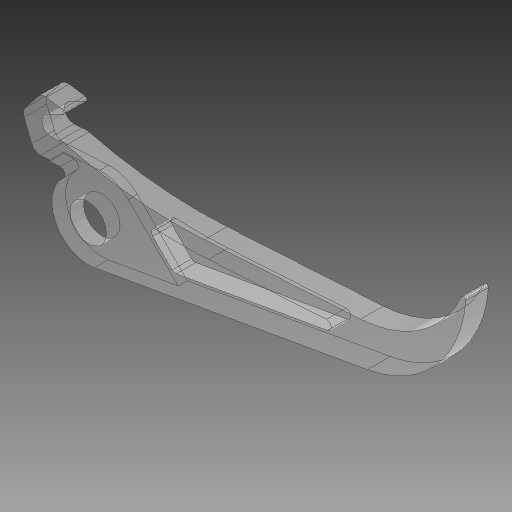
# Autodesk Inventor part: 後ウイング1.2
Saved by Autodesk Inventor 2020 (Build 240168000, 168)
## iProperties
Created: 2019-09-05
Part Number: 後ウイング1.2
Material: ポリカーボネート、クリア
Document SubType Name: Modeling
Designer: 雪村
Density: 1.2 g/cm^3
Appearance: ポリカーボネート - クリア
Mass: 5.3588 g
Surface Area: 38.9825 cm^2
Volume: 4.46567 cm^3
Description: ポリカ 5t
Author: 雪村
Autodesk Inventor part; units mm, degrees
ref_plane "YZ Plane" through (0, 0, 0) normal (1, 0, 0) x (0, 1, 0)
ref_plane "XZ Plane" through (0, 0, 0) normal (0, 1, 0) x (-1, 0, 0)
ref_plane "XY Plane" through (0, 0, 0) normal (0, 0, 1) x (1, 0, 0)
sketch "スケッチ1" plane through (0, 0, 0) normal (0, 0, 1) x (1, 0, 0)
  circle A0 centre (243.856358, 111.9666) radius 4.025
  circle A1 centre (243.856358, 111.9666) radius 8
  line L0 (245.245543, 104.088138) -> (305.438145, 114.701717)
  line L1 (243.379474, 119.952373) -> (303.875311, 123.564987)
  line L2 (243.856358, 111.9666) -> (322.640978, 125.858454) construction
  arc A2 (305.438145, 114.701717) -> (327.084101, 138.703402) centre (300.875427, 140.578172) ccw
  arc A3 (303.875311, 123.564987) -> (326.129046, 138.943438) centre (302.320232, 149.605909) ccw
  circle A4 centre (326.585375, 138.739077) radius 0.5
  line L3 (305.438145, 114.701717) -> (330.058338, 119.042922) construction
  line L4 (330.058338, 119.042922) -> (326.585375, 138.739077) construction
  line L5 (305.438145, 114.701717) -> (303.875311, 123.564987) construction
  point P0 (0, 0)
  point P1 (0, 0)
  dimension "d1" = 1
  dimension "d2" = 20
  dimension "d3" = 9
  dimension "d4" = 25
  dimension "d7" = 16
  dimension "d8" = 8.05
  constraints: 12 end point, 9 point on circle, 6 tangent, 5 centre point, 2 parallel, 2 perpendicular, 3 other
  measures "d1" diameter of A4
  measures "d2" distance of L3.end L4.end
  measures "d3" distance from line of L1.end L0
  measures "d4" distance of L0.end L3.end
  measures "d7" diameter of A1
  measures "d8" diameter of A0
extrude "押し出し1" add sketch "スケッチ1" along normal blind 5
sketch "スケッチ3" plane through (0, 0, 0) normal (0, 0, -1) x (-1, 0, 0)
  circle A0 centre (-243.856358, 111.9666) radius 4.025
  arc A1 (-326.129046, 138.943438) -> (-303.875311, 123.564987) centre (-302.320232, 149.605909) ccw
  arc A2 (-326.129046, 138.943438) -> (-327.084101, 138.703402) centre (-326.585375, 138.739077) ccw
  arc A3 (-327.084101, 138.703402) -> (-305.438145, 114.701717) centre (-300.875427, 140.578172) ccw
  line L0 (-245.245543, 104.088138) -> (-305.438145, 114.701717)
  arc A4 (-245.245543, 104.088138) -> (-243.379474, 119.952373) centre (-243.856358, 111.9666) ccw
  line L1 (-303.875311, 123.564987) -> (-243.379474, 119.952373)
  circle A5 centre (-243.856358, 111.9666) radius 4.025
  circle A6 centre (-243.856358, 111.9666) radius 8.25
  point P0 (0, 0)
  point P1 (-243.432312, 120.205695)
  point P2 (-245.288956, 103.841936)
  point P3 (-247.230487, 104.438137)
  point P4 (-245.391454, 120.072522)
  dimension "d9" = 16.5
  constraints: 1 centre point, 1 coincident
  measures "d9" diameter of A6
extrude "押し出し2" cut sketch "スケッチ3" against normal blind 2 contours A6 L0 A4 L1 | L1 A4 L0 A6
sketch "スケッチ4" plane through (0, 0, 5) normal (0, 0, 1) x (1, 0, 0)
  line L0 (303.875311, 123.564987) -> (245.391454, 120.072522)
  line L1 (245.391454, 120.072522) -> (235.409237, 119.476417)
  line L2 (235.409237, 119.476417) -> (235.051458, 125.467679)
  arc A0 (235.051458, 125.467679) -> (269.471333, 121.510494) centre (263.510279, 221.332665) ccw
  circle A1 centre (243.856358, 111.9666) radius 4.025
  circle A2 centre (237.755765, 122.120997) radius 2.5
  point P0 (0, 0)
  point P1 (0, 0)
  dimension "d44" = 5
  dimension "d45" = 100
  dimension "d46" = 10
  constraints: 4 end point, 4 tangent, 2 centre point, 2 point on circle, 1 collinear, 1 perpendicular, 1 point on line
  measures "d44" diameter of A2
  measures "d45" radius of A0
  measures "d46" distance of L0.end L1.end
extrude "押し出し3" add sketch "スケッチ4" against normal blind 5 contours L0 L1 A2 A0 | A2 L2 A0 | A2 | L1 L2 A2
sketch "スケッチ5" plane through (0, 0, 0) normal (0, 0, -1) x (-1, 0, 0)
  circle A0 centre (-243.856358, 111.9666) radius 4.025
  circle A1 centre (-243.856358, 111.9666) radius 8.25
  line L0 (-249.689989, 117.800231) -> (-288.164279, 79.32594)
  line L1 (-247.230487, 104.438137) -> (-305.438145, 114.701717)
  point P0 (0, 0)
  point P1 (-260.730499, 106.75972)
  point P2 (-245.288956, 103.841936)
  point P3 (-260.840494, 106.649726)
  point P4 (-260.680485, 106.809734)
  dimension "d35" = 16.5
  dimension "d36" = 55
  constraints: 2 end point, 1 centre point, 1 coincident, 1 point on circle, 1 tangent, 1 other
  measures "d35" diameter of A1
extrude "押し出し4" cut sketch "スケッチ5" against normal blind 2 contours A1 L1 L0
fillet "フィレット3" radius 3 1 edges at (235.0515, 125.4677, 2.5)
sketch "スケッチ6" plane through (0, 0, 5) normal (0, 0, 1) x (1, 0, 0)
  line L0 (245.391454, 120.072522) -> (243.379474, 119.952373)
  arc A0 (239.030137, 124.375341) -> (235.301068, 121.28779) centre (238.295733, 121.466622) ccw
  line L1 (235.301068, 121.28779) -> (235.409237, 119.476417)
  line L2 (235.409237, 119.476417) -> (243.379474, 119.952373)
  arc A1 (243.379474, 119.952373) -> (245.245543, 104.088138) centre (243.856358, 111.9666) ccw
  line L3 (245.245543, 104.088138) -> (305.438145, 114.701717)
  arc A2 (305.438145, 114.701717) -> (327.084101, 138.703402) centre (300.875427, 140.578172) ccw
  arc A3 (327.084101, 138.703402) -> (326.129046, 138.943438) centre (326.585375, 138.739077) ccw
  arc A4 (303.875311, 123.564987) -> (326.129046, 138.943438) centre (302.320232, 149.605909) ccw
  line L4 (303.875311, 123.564987) -> (269.471333, 121.510494)
  arc A5 (239.030137, 124.375341) -> (269.471333, 121.510494) centre (263.510279, 221.332665) ccw
  circle A6 centre (243.856358, 111.9666) radius 4.025
  circle A7 centre (237.79229, 118.616943) radius 1
  arc A8 (243.379474, 119.952373) -> (245.245543, 104.088138) centre (243.856358, 111.9666) ccw
  line L5 (235.409237, 119.476417) -> (243.379474, 119.952373)
  line L6 (235.301068, 121.28779) -> (235.409237, 119.476417)
  point P0 (0, 0)
  point P1 (236.794068, 118.557333)
  point P2 (238.466075, 117.878016)
  point P3 (237.732679, 119.615165)
  point P4 (237.732679, 119.615165)
  dimension "d55" = 2
  constraints: 5 other
extrude "押し出し5" add sketch "スケッチ6" against normal up to surface (3 mm away) contours A5 L4 A4 A3 A2 L3 A1 L2 L1 A0 | L2 A1 A7
sketch "スケッチ7" plane through (0, 0, 0) normal (0, 0, -1) x (-1, 0, 0)
  line L0 (-245.391454, 120.072522) -> (-235.409237, 119.476417)
  arc A0 (-245.391454, 120.072522) -> (-249.689989, 117.800231) centre (-243.856358, 111.9666) ccw
  line L1 (-260.680485, 106.809734) -> (-249.689989, 117.800231)
  circle A1 centre (-243.856358, 111.9666) radius 8.25
  line L2 (-243.364571, 120.201929) -> (-235.394334, 119.725972)
  line L3 (-235.409237, 119.476417) -> (-235.490786, 118.110823)
  arc A2 (-235.784063, 117.342881) -> (-236.275398, 114.521799) centre (-233.432538, 115.479999) ccw
  arc A3 (-238.466075, 117.878016) -> (-237.732679, 119.615165) centre (-237.79229, 118.616943) ccw
  line L4 (-235.409237, 119.476417) -> (-235.301068, 121.28779)
  point P0 (0, 0)
  point P1 (-249.689989, 117.800231)
  point P2 (-241.367494, 119.832224)
  dimension "d52" = 16.5
  constraints: 2 end point, 1 coincident, 1 parallel, 1 point on line, 4 other
extrude "押し出し6" cut sketch "スケッチ7" against normal blind 2 contours L0 A1 L2 L4 | A1 A0 L0 | L0 A1
sketch "スケッチ8" plane through (0, 0, 0) normal (0, 0, -1) x (-1, 0, 0)
  arc A0 (-243.364571, 120.201929) -> (-249.689989, 117.800231) centre (-243.856358, 111.9666) ccw
  line L0 (-243.364571, 120.201929) -> (-235.394334, 119.725972)
  line L1 (-235.394334, 119.725972) -> (-235.301068, 121.28779)
  arc A1 (-235.301068, 121.28779) -> (-239.030137, 124.375341) centre (-238.295733, 121.466622) ccw
  arc A2 (-269.471333, 121.510494) -> (-239.030137, 124.375341) centre (-263.510279, 221.332665) ccw
  line L2 (-303.875311, 123.564987) -> (-269.471333, 121.510494)
  arc A3 (-326.129046, 138.943438) -> (-303.875311, 123.564987) centre (-302.320232, 149.605909) ccw
  arc A4 (-326.129046, 138.943438) -> (-327.084101, 138.703402) centre (-326.585375, 138.739077) ccw
  arc A5 (-327.084101, 138.703402) -> (-305.438145, 114.701717) centre (-300.875427, 140.578172) ccw
  line L3 (-260.680485, 106.809734) -> (-305.438145, 114.701717)
  line L4 (-260.680485, 106.809734) -> (-249.689989, 117.800231)
  arc A6 (-235.68768, 124.269668) -> (-234.722388, 128.05367) centre (-235.624481, 126.268669) ccw
  line L5 (-232.816946, 130.554466) -> (-230.034777, 127.017584)
  arc A7 (-232.816946, 130.554466) -> (-234.673777, 131.297553) centre (-234.388893, 129.317947) ccw
  line L6 (-234.722388, 128.05367) -> (-238.29239, 129.857855)
  line L7 (-238.138088, 130.799007) -> (-234.673777, 131.297553)
  line L8 (-233.397891, 119.606751) -> (-235.394334, 119.725972)
  arc A8 (-233.397891, 119.606751) -> (-231.421838, 120.860108) centre (-233.27867, 121.603195) ccw
  line L9 (-229.749893, 125.037978) -> (-231.421838, 120.860108)
  arc A9 (-229.749893, 125.037978) -> (-230.034777, 127.017584) centre (-231.606724, 125.781065) ccw
  line L10 (-239.030137, 124.375341) -> (-235.68768, 124.269668)
  arc A10 (-238.138088, 130.799007) -> (-238.29239, 129.857855) centre (-238.066867, 130.304105) ccw
  line L11 (-235.394334, 119.725972) -> (-239.030137, 124.375341)
  line L12 (-235.394334, 119.725972) -> (-239.030137, 124.375341)
  arc A11 (-235.301068, 121.28779) -> (-239.030137, 124.375341) centre (-238.295733, 121.466622) ccw
  line L13 (-243.364571, 120.201929) -> (-235.394334, 119.725972)
  point P0 (0, 0)
  point P1 (-222.092413, 129.26267)
  point P2 (-237.379057, 124.323141)
  dimension "d56" = 2
  dimension "d57" = 2
  dimension "d58" = 4.5
  dimension "d59" = 2
  dimension "d60" = 4.5
  dimension "d61" = 2
  dimension "d62" = 3.5
  dimension "d63" = 0.5
  dimension "d64" = 4
  dimension "d65" = 2
  dimension "d66" = 25
  dimension "d67" = 35
  dimension "d68" = 120
  dimension "d69" = 120
  constraints: 16 end point, 11 tangent, 10 point on circle, 5 centre point
  measures "d56" distance of L0.end L8.start
  measures "d57" radius of A8
  measures "d58" distance of L9.start L9.end
  measures "d59" radius of A9
  measures "d60" distance of L5.start L5.end
  measures "d61" radius of A7
  measures "d62" distance of L7.start L7.end
  measures "d63" radius of A10
  measures "d64" distance of L6.start L6.end
  measures "d65" radius of A6
  measures "d66" angle of L6 L10
  measures "d67" angle of L7 L6
  measures "d68" angle of L7 L5
  measures "d69" angle of L9 L5
extrude "押し出し7" add sketch "スケッチ8" against normal blind 5 contours L1 A1 L10 A6 L6 A10 L7 A7 L5 A9 L9 A8 L8
shell "シェル1" thickness 4 removed faces 2 at (278.529988, 114.340648, 0) at (273.385007, 113.43345, 5)
fillet "フィレット5" radius 1 3 edges at (311.2887, 120.8864, 2.5) (255.5059, 117.6411, 2.5) (262.0365, 111.1105, 2.5)
sketch "スケッチ9" plane through (0, 0, 5) normal (0, 0, 1) x (1, 0, 0)
  arc A0 (258.140188, 117.471401) -> (269.709775, 117.517607) centre (263.510279, 221.332665) ccw
  line L0 (269.709775, 117.517607) -> (295.692908, 119.069235)
  arc A1 (295.926167, 117.086205) -> (295.692908, 119.069235) centre (295.752519, 118.071013) ccw
  line L1 (295.926167, 117.086205) -> (262.549185, 111.200943)
  arc A2 (261.66843, 111.478644) -> (262.549185, 111.200943) centre (262.375537, 112.185751) ccw
  line L2 (261.66843, 111.478644) -> (257.381445, 115.765628)
  arc A3 (258.140188, 117.471401) -> (257.381445, 115.765628) centre (258.088552, 116.472735) ccw
  line L3 (237.379057, 124.323141) -> (235.68768, 124.269668)
  arc A4 (234.722388, 128.05367) -> (235.68768, 124.269668) centre (235.624481, 126.268669) ccw
  line L4 (234.722388, 128.05367) -> (238.29239, 129.857855)
  arc A5 (238.29239, 129.857855) -> (238.138088, 130.799007) centre (238.066867, 130.304105) ccw
  line L5 (238.138088, 130.799007) -> (234.673777, 131.297553)
  arc A6 (234.673777, 131.297553) -> (232.816946, 130.554466) centre (234.388893, 129.317947) ccw
  line L6 (232.816946, 130.554466) -> (230.034777, 127.017584)
  arc A7 (230.034777, 127.017584) -> (229.749893, 125.037978) centre (231.606724, 125.781065) ccw
  line L7 (229.749893, 125.037978) -> (231.421838, 120.860108)
  arc A8 (231.421838, 120.860108) -> (233.397891, 119.606751) centre (233.27867, 121.603195) ccw
  line L8 (233.397891, 119.606751) -> (235.394334, 119.725972)
  line L9 (235.394334, 119.725972) -> (235.409237, 119.476417)
  line L10 (235.409237, 119.476417) -> (237.732679, 119.615165)
  arc A9 (238.466075, 117.878016) -> (237.732679, 119.615165) centre (237.79229, 118.616943) ccw
  arc A10 (238.466075, 117.878016) -> (245.245543, 104.088138) centre (243.856358, 111.9666) ccw
  line L11 (245.245543, 104.088138) -> (305.438145, 114.701717)
  arc A11 (305.438145, 114.701717) -> (327.084101, 138.703402) centre (300.875427, 140.578172) ccw
  arc A12 (327.084101, 138.703402) -> (326.129046, 138.943438) centre (326.585375, 138.739077) ccw
  arc A13 (303.875311, 123.564987) -> (326.129046, 138.943438) centre (302.320232, 149.605909) ccw
  line L12 (303.875311, 123.564987) -> (269.471333, 121.510494)
  arc A14 (239.030137, 124.375341) -> (269.471333, 121.510494) centre (263.510279, 221.332665) ccw
  arc A15 (239.030137, 124.375341) -> (237.379057, 124.323141) centre (238.295733, 121.466622) ccw
  circle A16 centre (243.856358, 111.9666) radius 4.025
  point P0 (0, 0)
extrude "押し出し8" add sketch "スケッチ9" against normal blind 0.7 contours A0 L0 A1 L1 A2 L2 A3
sketch "スケッチ10" plane through (0, 0, 0) normal (0, 0, -1) x (-1, 0, 0)
  line L0 (-243.364571, 120.201929) -> (-233.397891, 119.606751)
  arc A0 (-243.364571, 120.201929) -> (-249.689989, 117.800231) centre (-243.856358, 111.9666) ccw
  line L1 (-260.680485, 106.809734) -> (-249.689989, 117.800231)
  arc A1 (-261.066987, 106.423233) -> (-260.506855, 104.646723) centre (-260.324524, 105.680771) ccw
  arc A2 (-232.86586, 117.693214) -> (-233.397891, 119.606751) centre (-233.460482, 118.558618) ccw
  line L2 (-260.506855, 104.646723) -> (-245.610205, 102.020041)
  arc A3 (-245.610205, 102.020041) -> (-234.072915, 114.475431) centre (-243.856358, 111.9666) ccw
  line L3 (-261.066987, 106.423233) -> (-260.680485, 106.809734)
  arc A4 (-232.86586, 117.693214) -> (-234.072915, 114.475431) centre (-231.166941, 115.220629) ccw
  line L4 (-295.692908, 119.069235) -> (-269.709775, 117.517607)
  arc A5 (-295.692908, 119.069235) -> (-295.926167, 117.086205) centre (-295.752519, 118.071013) ccw
  line L5 (-262.549185, 111.200943) -> (-295.926167, 117.086205)
  arc A6 (-262.549185, 111.200943) -> (-261.66843, 111.478644) centre (-262.375537, 112.185751) ccw
  line L6 (-257.381445, 115.765628) -> (-261.66843, 111.478644)
  arc A7 (-257.381445, 115.765628) -> (-258.140188, 117.471401) centre (-258.088552, 116.472735) ccw
  arc A8 (-269.709775, 117.517607) -> (-258.140188, 117.471401) centre (-263.510279, 221.332665) ccw
  line L7 (-237.379057, 124.323141) -> (-235.68768, 124.269668)
  arc A9 (-235.68768, 124.269668) -> (-234.722388, 128.05367) centre (-235.624481, 126.268669) ccw
  line L8 (-234.722388, 128.05367) -> (-238.29239, 129.857855)
  arc A10 (-238.138088, 130.799007) -> (-238.29239, 129.857855) centre (-238.066867, 130.304105) ccw
  line L9 (-238.138088, 130.799007) -> (-234.673777, 131.297553)
  arc A11 (-232.816946, 130.554466) -> (-234.673777, 131.297553) centre (-234.388893, 129.317947) ccw
  line L10 (-232.816946, 130.554466) -> (-230.034777, 127.017584)
  arc A12 (-229.749893, 125.037978) -> (-230.034777, 127.017584) centre (-231.606724, 125.781065) ccw
  line L11 (-229.749893, 125.037978) -> (-231.421838, 120.860108)
  arc A13 (-233.397891, 119.606751) -> (-231.421838, 120.860108) centre (-233.27867, 121.603195) ccw
  line L12 (-233.397891, 119.606751) -> (-235.394334, 119.725972)
  line L13 (-235.394334, 119.725972) -> (-235.409237, 119.476417)
  line L14 (-235.409237, 119.476417) -> (-237.732679, 119.615165)
  arc A14 (-237.732679, 119.615165) -> (-238.466075, 117.878016) centre (-237.79229, 118.616943) ccw
  arc A15 (-245.245543, 104.088138) -> (-238.466075, 117.878016) centre (-243.856358, 111.9666) ccw
  line L15 (-245.245543, 104.088138) -> (-305.438145, 114.701717)
  arc A16 (-327.084101, 138.703402) -> (-305.438145, 114.701717) centre (-300.875427, 140.578172) ccw
  arc A17 (-326.129046, 138.943438) -> (-327.084101, 138.703402) centre (-326.585375, 138.739077) ccw
  arc A18 (-326.129046, 138.943438) -> (-303.875311, 123.564987) centre (-302.320232, 149.605909) ccw
  line L16 (-303.875311, 123.564987) -> (-269.471333, 121.510494)
  arc A19 (-269.471333, 121.510494) -> (-239.030137, 124.375341) centre (-263.510279, 221.332665) ccw
  arc A20 (-237.379057, 124.323141) -> (-239.030137, 124.375341) centre (-238.295733, 121.466622) ccw
  circle A21 centre (-243.856358, 111.9666) radius 4.025
  point P0 (0, 0)
  dimension "d77" = 2.1
  dimension "d78" = 2.1
  dimension "d80" = 3
  constraints: 8 point on circle, 6 tangent, 5 end point, 4 centre point, 2 other
  measures "d77" diameter of A1
  measures "d78" diameter of A2
  measures "d80" radius of A4
